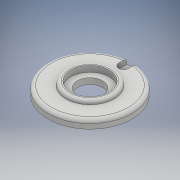
# Autodesk Inventor part: 도면3-2번
Saved by Autodesk Inventor 2018.3 (Build 223284000, 284)
## iProperties
Created: 2019-10-10
Part Number: 도면3-2번
Material: 일반
Document SubType Name: Modeling
Designer: MyTool
Density: 1 g/cm^3
Appearance: 기본값
Author: MyTool
Autodesk Inventor part; units mm, degrees
ref_plane "YZ Plane" through (0, 0, 0) normal (1, 0, 0) x (0, 1, 0)
ref_plane "XZ Plane" through (0, 0, 0) normal (0, 1, 0) x (-1, 0, 0)
ref_plane "XY Plane" through (0, 0, 0) normal (0, 0, 1) x (1, 0, 0)
sketch "스케치13" plane through (0, 0, 0) normal (0, 0, 1) x (1, 0, 0)
  circle A0 centre (0, 0) radius 35
  dimension "d74" = 70
  constraints: 1 centre point, 1 coincident
  measures "d74" diameter of A0
extrude "돌출11" add sketch "스케치13" along normal blind 7
sketch "스케치19" plane through (0, 0, 7) normal (0, 0, 1) x (1, 0, 0)
  circle A0 centre (0, 0) radius 20
  dimension "d92" = 40
  constraints: 1 centre point, 1 coincident
  measures "d92" diameter of A0
extrude "돌출17" add sketch "스케치19" along normal blind 3
sketch "스케치20" plane through (0, 0, 10) normal (0, 0, 1) x (1, 0, 0)
  circle A0 centre (0, 0) radius 16
  dimension "d95" = 32
  constraints: 1 centre point, 1 coincident
  measures "d95" diameter of A0
extrude "돌출18" cut sketch "스케치20" against normal blind 5
sketch "스케치16" plane through (0, 0, 0) normal (0, 0, -1) x (-1, 0, 0)
  circle A0 centre (0, 0) radius 23.5
  dimension "d83" = 47
  constraints: 1 centre point, 1 coincident
  measures "d83" diameter of A0
extrude "돌출15" add sketch "스케치16" along normal blind 3
sketch "스케치23" plane through (0, 0, -3) normal (0, 0, -1) x (-1, 0, 0)
  circle A0 centre (0, 0) radius 18.5
  dimension "d117" = 37
  constraints: 1 centre point, 1 coincident
  measures "d117" diameter of A0
extrude "돌출20" cut sketch "스케치23" against normal blind 3
sketch "스케치18" plane through (0, 0, -3) normal (0, 0, -1) x (-1, 0, 0)
  circle A0 centre (0, 0) radius 10.5
  dimension "d89" = 21
  constraints: 1 centre point, 1 coincident
  measures "d89" diameter of A0
extrude "돌출16" cut sketch "스케치18" against normal up to next
sketch "스케치21" plane through (0, 0, 7) normal (0, 0, 1) x (1, 0, 0)
  circle A0 centre (0, 28) radius 4
  line L0 (-4, 28) -> (4, 28)
  line L1 (4, 28) -> (4, 38)
  line L2 (4, 38) -> (-4, 38)
  line L3 (-4, 38) -> (-4, 28)
  point P0 (0, 0)
  dimension "d99" = 8
  dimension "d100" = 28
  constraints: 8 end point, 2 parallel, 2 point on circle, 1 centre point, 1 horizontal, 1 perpendicular
  measures "d99" diameter of A0
  measures "d100" distance of point (0, 0) A0.centre
extrude "돌출19" cut sketch "스케치21" against normal blind 4.4
sketch "스케치22" plane through (0, 0, 2.6) normal (0, 0, 1) x (1, 0, 0)
  arc A0 (-4, 28) -> (4, 28) centre (0, 28) ccw projected
  circle A1 centre (0, 28) radius 4
  point P0 (0, 0)
  constraints: 1 centre point, 1 coincident
hole "구멍2" at (0, 28, 2.6) direction (0, 0, -1) diameter 4.5 end through all
fillet "모깎기7" radius 3 4 edges at (-23.2916, -26.1247, 7) (26.1247, 23.2916, 7) (-20, 0, 10) (18.5, 0, 0)
chamfer "모따기6" distance 1 angle 45 1 edges at (23.5, 0, -3)
